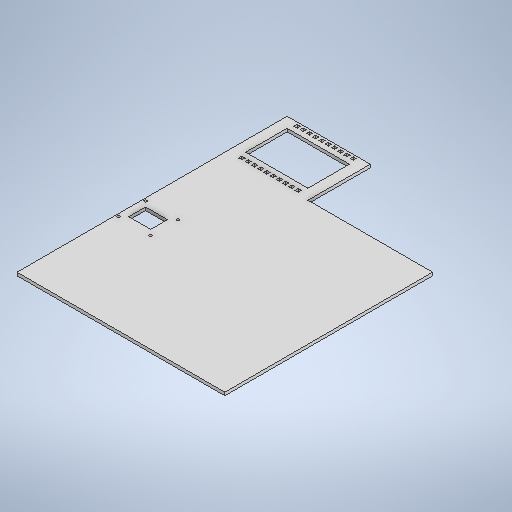
# Autodesk Inventor part: base zzzz
Saved by Autodesk Inventor 2025.3 (Build 293356000, 356)
## iProperties
Created: 2026-05-01
Part Number: base zzzz
Material: Generic
Document SubType Name: Modeling
Designer: kamal
Density: 1 g/cm^3
Appearance: Default
Author: kamal
Autodesk Inventor part; units mm, degrees
ref_plane "YZ Plane" through (0, 0, 0) normal (1, 0, 0) x (0, 1, 0)
ref_plane "XZ Plane" through (0, 0, 0) normal (0, 1, 0) x (-1, 0, 0)
ref_plane "XY Plane" through (0, 0, 0) normal (0, 0, 1) x (1, 0, 0)
sketch "Sketch1" plane through (0, 0, 0) normal (0, 1, 0) x (-1, 0, 0)
  line L0 (-200, 200) -> (200, 200)
  line L1 (200, 200) -> (200, -200)
  line L2 (200, -200) -> (-200, -200)
  line L3 (-200, -200) -> (-200, 200)
  line L4 (-200, 200) -> (200, -200) construction
  line L5 (200, 200) -> (-200, -200) construction
  point P0 (0, 0)
  dimension "d0" = 400
  dimension "d1" = 400
  constraints: 12 end point, 2 midpoint, 2 parallel, 1 horizontal, 1 perpendicular
  measures "d0" distance of L1.end L2.end
  measures "d1" distance of L0.end L1.end
extrude "Extrusion1" add sketch "Sketch1" along normal blind 6
sketch "Sketch2" plane through (0, 6, 0) normal (0, 1, 0) x (1, 0, 0)
  line L0 (-190, -5) -> (-137.7238, -5)
  line L1 (-137.7238, -5) -> (-137.7238, 37.4)
  line L2 (-190, 37.4) -> (-137.7238, 37.4)
  line L3 (-190, -5) -> (-190, 37.4)
  line L4 (-142.7238, 32.4) -> (-142.7238, 0)
  line L5 (-142.7238, 0) -> (-185, 0)
  line L6 (-185, 0) -> (-185, 32.4)
  line L7 (-185, 32.4) -> (-142.7238, 32.4)
  line L8 (-127.7238, 47.4) -> (-127.7238, -15)
  line L9 (-127.7238, -15) -> (-200, -15)
  line L10 (-200, -15) -> (-200, 47.4)
  line L11 (-200, 47.4) -> (-127.7238, 47.4)
  line L12 (-132.7238, 42.4) -> (-132.7238, -10) construction
  line L13 (-132.7238, -10) -> (-195, -10) construction
  line L14 (-195, -10) -> (-195, 42.4) construction
  line L15 (-195, 42.4) -> (-132.7238, 42.4) construction
  circle A0 centre (-132.7238, 42.4) radius 2.5
  circle A1 centre (-195, 42.4) radius 2.5
  circle A2 centre (-195, -10) radius 2.5
  circle A3 centre (-132.7238, -10) radius 2.5
  line L16 (-200, -200) -> (200, -200) projected
  line L17 (-200, 200) -> (-200, -200) projected
  point P0 (0, 0)
  point P1 (-163.8619, -15)
  dimension "d4" = 5
  dimension "d5" = 10
  dimension "d6" = 5
  dimension "d7" = 5
  dimension "d8" = 5
  dimension "d9" = 5
  dimension "d10" = 5
  dimension "d11" = 62.4
  dimension "d12" = 72.2762
  dimension "d13" = 42.4
  dimension "d14" = 52.2762
  dimension "d18" = 185
  constraints: 32 end point, 4 centre point, 4 coincident, 1 collinear, 1 midpoint, 1 parallel, 9 other
  measures "d4" distance between parallel lines of L1 L4
  measures "d5" distance between parallel lines of L1 L8
  measures "d6" distance between parallel lines of L1 L12
  measures "d7" diameter of A0
  measures "d8" diameter of A1
  measures "d9" diameter of A2
  measures "d10" diameter of A3
  measures "d11" distance of L9.end L11.start
  measures "d12" distance of L11.start L11.end
  measures "d13" distance of L0.start L2.start
  measures "d14" distance of L2.start L2.end
  measures "d18" distance from line of point (-163.862, -15) L16
extrude "Extrusion2" cut sketch "Sketch2" against normal through all contours L4 L5 L6 L7 | A0 | A1 | A2 | A3
sketch "Sketch3" plane through (0, 6, 0) normal (0, 1, 0) x (1, 0, 0)
  line L0 (200, 200) -> (-200, 200) projected
  line L1 (-200, 200) -> (-200, 320)
  line L2 (-200, 320) -> (-40, 320)
  line L3 (-40, 320) -> (-40, 200)
  line L4 (-180, 300) -> (-60, 300)
  line L5 (-60, 300) -> (-60, 220)
  line L6 (-60, 220) -> (-180, 220)
  line L7 (-180, 220) -> (-180, 300)
  point P0 (0, 0)
  point P1 (-120, 300)
  dimension "d19" = 120
  dimension "d20" = 160
  dimension "d21" = 120
  dimension "d22" = 80
  dimension "d23" = 20
  dimension "d24" = 20
  constraints: 14 end point, 2 horizontal, 2 parallel, 2 perpendicular, 1 midpoint, 1 point on line, 1 vertical
  measures "d19" distance of L0.end L1.end
  measures "d20" distance of L1.end L2.end
  measures "d21" distance of L5.end L6.end
  measures "d22" distance of L4.end L5.end
  measures "d23" distance from line of point (-120, 300) L2
  measures "d24" distance between parallel lines of L1 L7
extrude "Extrusion3" add sketch "Sketch3" against normal blind 6
sketch "Sketch4" plane through (0, 6, 0) normal (0, 1, 0) x (1, 0, 0)
  line L0 (-180, 210) -> (-60, 210)
  line L1 (-60, 210) -> (-60, 204)
  line L2 (-60, 204) -> (-180, 204)
  line L3 (-180, 204) -> (-180, 210)
  line L4 (-60, 220) -> (-180, 220) projected
  line L5 (-200, 320) -> (-200, -200) projected
  line L6 (-177, 210) -> (-177, 204)
  line L7 (-171, 210) -> (-171, 204)
  line L8 (-171, 210) -> (-171, 204)
  line L9 (-165, 210) -> (-165, 204)
  line L10 (-165, 210) -> (-165, 204)
  line L11 (-159, 210) -> (-159, 204)
  line L12 (-159, 210) -> (-159, 204)
  line L13 (-153, 210) -> (-153, 204)
  line L14 (-153, 210) -> (-153, 204)
  line L15 (-147, 210) -> (-147, 204)
  line L16 (-147, 210) -> (-147, 204)
  line L17 (-141, 210) -> (-141, 204)
  line L18 (-141, 210) -> (-141, 204)
  line L19 (-135, 210) -> (-135, 204)
  line L20 (-135, 210) -> (-135, 204)
  line L21 (-129, 210) -> (-129, 204)
  line L22 (-129, 210) -> (-129, 204)
  line L23 (-123, 210) -> (-123, 204)
  line L24 (-123, 210) -> (-123, 204)
  line L25 (-117, 210) -> (-117, 204)
  line L26 (-117, 210) -> (-117, 204)
  line L27 (-111, 210) -> (-111, 204)
  line L28 (-111, 210) -> (-111, 204)
  line L29 (-105, 210) -> (-105, 204)
  line L30 (-105, 210) -> (-105, 204)
  line L31 (-99, 210) -> (-99, 204)
  line L32 (-99, 210) -> (-99, 204)
  line L33 (-93, 210) -> (-93, 204)
  line L34 (-93, 210) -> (-93, 204)
  line L35 (-87, 210) -> (-87, 204)
  line L36 (-87, 210) -> (-87, 204)
  line L37 (-81, 210) -> (-81, 204)
  line L38 (-81, 210) -> (-81, 204)
  line L39 (-75, 210) -> (-75, 204)
  line L40 (-75, 210) -> (-75, 204)
  line L41 (-69, 210) -> (-69, 204)
  line L42 (-69, 210) -> (-69, 204)
  line L43 (-63, 210) -> (-63, 204)
  line L44 (-180, 220) -> (-180, 300) projected
  line L45 (-180, 300) -> (-60, 300) projected
  line L46 (-60, 300) -> (-60, 220) projected
  line L47 (-180, 260) -> (-60, 260) construction
  line L48 (-180, 310) -> (-60, 310)
  line L49 (-60, 310) -> (-60, 316)
  line L50 (-60, 316) -> (-180, 316)
  line L51 (-180, 316) -> (-180, 310)
  line L52 (-177, 310) -> (-177, 316)
  line L53 (-171, 310) -> (-171, 316)
  line L54 (-171, 310) -> (-171, 316)
  line L55 (-165, 310) -> (-165, 316)
  line L56 (-165, 310) -> (-165, 316)
  line L57 (-159, 310) -> (-159, 316)
  line L58 (-159, 310) -> (-159, 316)
  line L59 (-153, 310) -> (-153, 316)
  line L60 (-153, 310) -> (-153, 316)
  line L61 (-147, 310) -> (-147, 316)
  line L62 (-147, 310) -> (-147, 316)
  line L63 (-141, 310) -> (-141, 316)
  line L64 (-141, 310) -> (-141, 316)
  line L65 (-135, 310) -> (-135, 316)
  line L66 (-135, 310) -> (-135, 316)
  line L67 (-129, 310) -> (-129, 316)
  line L68 (-129, 310) -> (-129, 316)
  line L69 (-123, 310) -> (-123, 316)
  line L70 (-123, 310) -> (-123, 316)
  line L71 (-117, 310) -> (-117, 316)
  line L72 (-117, 310) -> (-117, 316)
  line L73 (-111, 310) -> (-111, 316)
  line L74 (-111, 310) -> (-111, 316)
  line L75 (-105, 310) -> (-105, 316)
  line L76 (-105, 310) -> (-105, 316)
  line L77 (-99, 310) -> (-99, 316)
  line L78 (-99, 310) -> (-99, 316)
  line L79 (-93, 310) -> (-93, 316)
  line L80 (-93, 310) -> (-93, 316)
  line L81 (-87, 310) -> (-87, 316)
  line L82 (-87, 310) -> (-87, 316)
  line L83 (-81, 310) -> (-81, 316)
  line L84 (-81, 310) -> (-81, 316)
  line L85 (-75, 310) -> (-75, 316)
  line L86 (-75, 310) -> (-75, 316)
  line L87 (-69, 310) -> (-69, 316)
  line L88 (-69, 310) -> (-69, 316)
  line L89 (-63, 310) -> (-63, 316)
  point P0 (0, 0)
  point P1 (-180, 207)
  point P2 (-177, 207)
  point P3 (-171, 207)
  point P4 (-165, 207)
  point P5 (-159, 207)
  point P6 (-153, 207)
  point P7 (-147, 207)
  point P8 (-141, 207)
  point P9 (-135, 207)
  point P10 (-129, 207)
  point P11 (-123, 207)
  point P12 (-117, 207)
  point P13 (-111, 207)
  point P14 (-105, 207)
  point P15 (-99, 207)
  point P16 (-93, 207)
  point P17 (-87, 207)
  point P18 (-81, 207)
  point P19 (-75, 207)
  point P20 (-69, 207)
  point P21 (-180, 313)
  point P22 (-177, 313)
  point P23 (-171, 313)
  point P24 (-165, 313)
  point P25 (-159, 313)
  point P26 (-153, 313)
  point P27 (-147, 313)
  point P28 (-141, 313)
  point P29 (-135, 313)
  point P30 (-129, 313)
  point P31 (-123, 313)
  point P32 (-117, 313)
  point P33 (-111, 313)
  point P34 (-105, 313)
  point P35 (-99, 313)
  point P36 (-93, 313)
  point P37 (-87, 313)
  point P38 (-81, 313)
  point P39 (-75, 313)
  point P40 (-69, 313)
  dimension "d27" = 120
  dimension "d28" = 6
  dimension "d29" = 10
  dimension "d30" = 20
  dimension "d31" = 3
  dimension "d32" = 6
  dimension "d35" = 6
  constraints: 162 end point, 100 symmetric about line, 90 horizontal alignment, 37 parallel, 4 midpoint, 3 vertical, 20 other
  measures "d27" distance of L1.end L3.start
  measures "d28" distance of L1.start L1.end
  measures "d30" distance from line of L5 point (-180, 207)
  measures "d31" distance of point (-180, 207) point (-177, 207)
  measures "d32" distance between parallel lines of L7 L6
  measures "d35" distance of L6.start L8.start
extrude "Extrusion4" cut sketch "Sketch4" against normal blind 6 contours L0 L7 L2 L6 | L0 L11 L2 L9 | L0 L15 L2 L13 | L0 L19 L2 L17 | L0 L23 L2 L21 | L0 L27 L2 L25 | L0 L31 L2 L29 | L0 L35 L2 L33 | L0 L39 L2 L37 | L0 L43 L2 L41 | L52 L50 L53 L48 | L55 L50 L57 L48 | L59 L50 L61 L48 | L63 L50 L65 L48 | L67 L50 L69 L48 | L71 L50 L73 L48 | L75 L50 L77 L48 | L79 L50 L81 L48 | L83 L50 L85 L48 | L87 L50 L89 L48
sketch "Sketch5" plane through (0, 6, 0) normal (0, 1, 0) x (1, 0, 0)
  line L0 (200, -200) -> (200, 200) projected
  line L1 (200, 200) -> (-40, 200) projected
  line L2 (200, 0) -> (-40, 0)
  line L3 (-40, 0) -> (-40, 200)
  line L4 (-40, 200) -> (200, 200)
  line L5 (200, 200) -> (200, 0)
  point P0 (0, 0)
  dimension "d42" = 240
  constraints: 8 end point, 2 parallel, 1 horizontal, 1 midpoint, 1 perpendicular, 1 point on line
  measures "d42" distance between parallel lines of L0 L3
equation "\"d40\" = d32"
body "Solid1"
